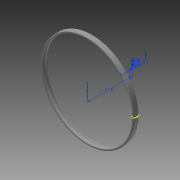
# Autodesk Inventor part: TyreDia120mm
Saved by Autodesk Inventor 2014 SP1 (Build 180222100, 222)
## iProperties
Created: 2017-01-08
Part Number: TyreDia120mm
Material: Generic
Document SubType Name: Modeling
Designer: danielsikar
Density: 1 g/cm^3
Appearance: White
Author: danielsikar
Autodesk Inventor part; units mm, degrees
ref_plane "XZ Plane" through (0, 0, 0) normal (0, 1, 0) x (-1, 0, 0)
ref_plane "XY Plane" through (0, 0, 0) normal (0, 0, 1) x (1, 0, 0)
sketch "Sketch2" plane through (0, 0, 0) normal (0, 0, 1) x (1, 0, 0)
  line L0 (53.3149, 0) -> (65.6581, 0) construction
  line L1 (52.1637, 6.5) -> (72.8804, 6.5) construction
  line L2 (57.5, 7.9191) -> (57.5, -2.7391) construction
  line L3 (56.8, 7.9191) -> (56.8, -5.2764) construction
  line L4 (58.2, 7.9191) -> (58.2, -2.2873) construction
  line L5 (54.0761, 3.25) -> (61.4731, 3.25) construction
  arc A0 (57.5321, 5.338) -> (57.5321, 1.162) centre (60.1406, 3.25) ccw
  arc A1 (57.5321, 5.338) -> (57.5, 6.5) centre (56.83, 5.9) ccw
  arc A2 (57.5, 0) -> (57.5321, 1.162) centre (56.83, 0.6) ccw
  line L6 (57.5, 0) -> (59.3708, 0)
  line L7 (59.3708, 0) -> (59.3708, 6.5)
  line L8 (59.3708, 6.5) -> (57.5, 6.5)
  line L9 (57.5, 6.5) -> (59.3708, 6.5)
  line L10 (57.5, 0) -> (59.3708, 0)
  line L11 (59.3708, 6.5) -> (59.3708, 0)
  line L12 (0, -7.9156) -> (0, 10.5583) projected
  point P0 (0, 0)
  dimension "d0" = 6.5
  dimension "d1" = 57.5
  dimension "d2" = 0.7
  dimension "d3" = 0.7
  dimension "d4" = 3.25
  constraints: 24 end point, 10 point on circle, 5 point on line, 3 centre point, 1 horizontal, 1 parallel, 1 perpendicular, 3 other
  measures "d0" distance between parallel lines of L1 L0
  measures "d1" distance from line of L2 point (0, 0)
  measures "d2" distance from line of L2.end L3
  measures "d3" distance between parallel lines of L4 L2
  measures "d4" distance between parallel lines of L0 L5
revolve "Revolution1" add sketch "Sketch2" angle 360 about axis through (0, -10, 0) along (0, 1, 0)
chamfer "Chamfer1" distance 0.5 angle 45 2 edges at (-59.3708, 6.5, 0) (-59.3708, 0, 0)
ref_plane "Work Plane1" through (60, 0, 0) normal (1, 0, 0) x (0, 1, 0)
sketch "Sketch4" plane through (60, 0, 0) normal (1, 0, 0) x (0, 1, 0)
  line L0 (3.25, 2.7887) -> (3.25, -7.2593) construction
  line L1 (1, 2.7887) -> (3.25, -2.8543)
  line L2 (3.25, -2.8543) -> (5.5, 2.7887)
  line L3 (4.0887, 3.6948) -> (4.0887, -0.6025) construction
  line L4 (4.0887, 3.6948) -> (8.386, 3.6948) construction
  line L5 (2.25, 2.7887) -> (3.25, 0.4138)
  line L6 (3.25, 0.4138) -> (4.25, 2.7887)
  line L7 (1, 2.7887) -> (2.25, 2.7887)
  line L8 (4.25, 2.7887) -> (5.5, 2.7887)
  line L9 (2.5335, 3.6948) -> (2.5335, 2.7887) construction
  line L10 (2.5335, 2.1155) -> (2.5335, -0.3536) construction
  line L11 (4.25, 2.7887) -> (3.25, 0.4138)
  line L12 (2.25, 2.7887) -> (3.25, 0.4138)
  line L13 (1, 2.7887) -> (3.2549, -2.8665)
  line L14 (5.5001, 2.7887) -> (3.25, -2.8788)
  line L15 (5.5001, 2.7887) -> (4.25, 2.7887)
  line L16 (2.25, 2.7887) -> (1, 2.7887)
  point P0 (0, 0)
  dimension "d18" = 90
  constraints: 34 end point, 5 point on line, 3 horizontal, 1 perpendicular
  measures "d18" angle of L3 L4
extrude "Extrusion1" add sketch "Sketch4" against normal up to surface contours L7 L5 L6 L8 L2 L1
chamfer "Chamfer2" distance 0.2 angle 45 6 edges at (60, 1.625, 2.7887) (60, 2.75, 1.6013) (60, 3.75, 1.6013) (60, 4.875, 2.7887) (60, 4.375, -0.0328) (60, 2.125, -0.0328)
pattern_circular "Circular Pattern1" count 56 over 360 about axis through (0, -10, 0) along (0, 1, 0) of "Extrusion1"
body "Solid1"
